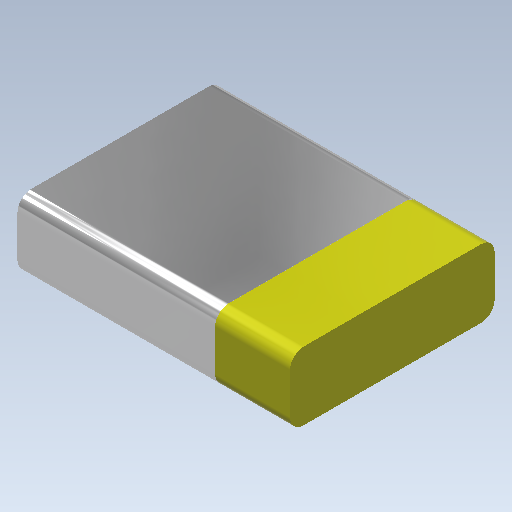
# Autodesk Inventor part: bateria litio
Saved by Autodesk Inventor 2020 (Build 240168000, 168)
## iProperties
Created: 2020-11-11
Part Number: bateria litio
Material: Genérico
Document SubType Name: Modeling
Designer: itala
Density: 1 g/cm^3
Appearance: Aluminio - Plano
Mass: 1.48283 g
Surface Area: 10.6223 cm^2
Volume: 1.48283 cm^3
Author: itala
Autodesk Inventor part; units mm, degrees
ref_plane "YZ Plane" through (0, 0, 0) normal (1, 0, 0) x (0, 1, 0)
ref_plane "XZ Plane" through (0, 0, 0) normal (0, 1, 0) x (-1, 0, 0)
sketch "Boceto1" plane through (0, 0, 0) normal (0, 1, 0) x (-1, 0, 0)
  line L0 (9.0859, 5.6094) -> (-10.9141, 5.6094)
  line L1 (-10.9141, 5.6094) -> (-10.9141, -9.3906)
  line L2 (-10.9141, -9.3906) -> (9.0859, -9.3906)
  line L3 (9.0859, -9.3906) -> (9.0859, 5.6094)
  point P0 (0, 0)
  dimension "d0" = 20
  dimension "d1" = 15
  constraints: 8 end point, 2 parallel, 1 horizontal, 1 perpendicular
  measures "d0" distance of L1.end L2.end
  measures "d1" distance of L0.end L1.end
extrude "Extrusión1" add sketch "Boceto1" along normal blind 5
ref_plane "Plano de trabajo1" through (5.4141, 0, 5.6094) normal (1, 0, 0) x (0, 0, -1)
split body "Dividir1" result two bodies by plane through (5.4141, 0, 5.6094) normal (1, 0, 0) first body at (9.0808, 0.5, 0.6094)
fillet "Empalme1" radius 1 8 edges at (8.1641, 5, -9.3906) (8.1641, 0, -9.3906) (8.1641, 5, 5.6094) (8.1641, 0, 5.6094) (-1.8359, 5, -9.3906) (-1.8359, 0, -9.3906) (-1.8359, 5, 5.6094) (-1.8359, 0, 5.6094)
